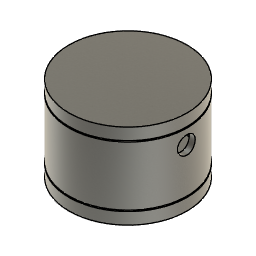
prototipo1 v3 (Autodesk Fusion 360 design; units mm, degrees)
Autodesk Fusion 360 part; units mm, degrees
note: some values were not read from the file. Chosen so that the rebuilt part matches the saved one: where a step ends.
sketch "Boceto1" plane through (0, 0, 0) normal (0, 0, 1) x (1, 0, 0)
  circle A0 centre (0, 0) radius 50
  circle A1 centre (0, 0) radius 45
  dimension "d1" = 100
  dimension "d2" = 90
  constraint coincident A0.centre A1.centre
  measures "d1" diameter of A0
  measures "d2" diameter of A1
extrude "Extruir1" add sketch "Boceto1" along normal blind 50 makes body 1
ref_plane "PlanoDeObra1" through (0, 0, 51) normal (0, 0, 1) x (1, 0, 0)
sketch "Boceto3" plane through (0, 0, 51) normal (0, 0, 1) x (1, 0, 0)
  circle A0 centre (0, 0) radius 50
  dimension "d6" = 100
  constraint coincident A0.centre origin
  measures "d6" diameter of A0
extrude "Extruir2" add sketch "Boceto3" along normal blind 10 separate body makes body 2
ref_plane "PlanoDeObra2" through (0, 0, -1) normal (0, 0, -1) x (-1, 0, 0)
sketch "Boceto4" plane through (0, 0, -1) normal (0, 0, -1) x (1, 0, 0)
  circle A0 centre (0, 0) radius 50
  dimension "d10" = 100
  constraint coincident A0.centre origin
  measures "d10" diameter of A0
extrude "Extruir3" add sketch "Boceto4" along normal blind 10 separate body makes body 3
sketch "Boceto5" plane through (0, 0, -11) normal (0, 0, -1) x (1, 0, 0)
  circle A0 centre (0, 0) radius 50
  line L0 (-25, 25) -> (25, 25)
  line L1 (25, 25) -> (25, -25)
  line L2 (25, -25) -> (-25, -25)
  line L3 (-25, -25) -> (-25, 25)
  dimension "d13" = 50
  dimension "d14" = 25
  dimension "d15" = 50
  dimension "d16" = 25
  constraint horizontal L0
  constraint vertical L1
  constraint horizontal L2
  constraint vertical L3
  measures "d13" distance of L0.start L0.end
  measures "d14" distance of A0.centre L1
  measures "d15" distance of L0.end L1.end
  measures "d16" distance of A0.centre L2
extrude "Extruir4" cut sketch "Boceto5" along normal up to far side of body 3 contours L0 L1 L2 L3 bodies 3
ref_plane "PlanoDeObra3" through (50, 0, 20.0968) normal (1, 0, 0) x (0, -1, 0)
sketch "Boceto6" plane through (50, 0, 20.0968) normal (1, 0, 0) x (0, 1, 0)
  line L0 (-50, 30) -> (50, 30)
  line L1 (50, 30) -> (50, -20)
  line L2 (50, -20) -> (-50, -20)
  line L3 (-50, -20) -> (-50, 30)
  circle A0 centre (0, 17.5) radius 7.5
  dimension "d20" = 15
  dimension "d21" = 12.5
  dimension "d22" = 100
  dimension "d23" = 50
  dimension "d24" = 20
  dimension "d25" = 50
  dimension "d26" = 50
  constraint horizontal L0
  constraint vertical L1
  constraint horizontal L2
  constraint vertical L3
  measures "d20" diameter of A0
  measures "d21" distance of L0 A0.centre
  measures "d22" distance of L1.end L2.end
  measures "d23" distance of L0.end L1.end
  measures "d24" vertical distance of origin L1.end
  measures "d25" distance of origin L1
  measures "d26" distance of L3 A0.centre
hole "Agujero1" at (50, 0, 37.5968) direction (-1, 0, 0) diameter 15 end through all bodies 1
equation "d21 = 5 mm + 7.5 mm"
